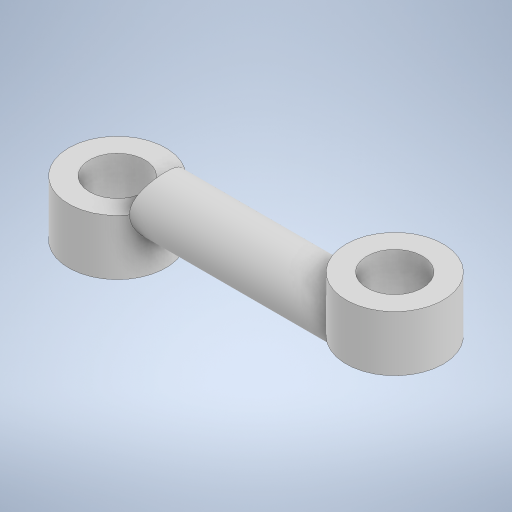
# Autodesk Inventor part: Part3
Saved by Autodesk Inventor 2024 (Build 280153000, 153)
## iProperties
Created: 2023-10-11
Part Number: Part3
Material: Generic
Document SubType Name: Modeling
Designer: owner
Density: 1 g/cm^3
Appearance: Default
Author: owner
Autodesk Inventor part; units mm, degrees
ref_plane "YZ Plane" through (0, 0, 0) normal (1, 0, 0) x (0, 1, 0)
ref_plane "XZ Plane" through (0, 0, 0) normal (0, 1, 0) x (-1, 0, 0)
ref_plane "XY Plane" through (0, 0, 0) normal (0, 0, 1) x (1, 0, 0)
sketch "Sketch1" plane through (0, 0, 0) normal (0, 0, 1) x (1, 0, 0)
  line L0 (-50, 0) -> (50, 0)
  line L1 (0, 0) -> (0, 34.9563) construction
  line L2 (-50, 0) -> (-50, 10)
  line L3 (-50, 10) -> (50, 10)
  line L4 (50, 10) -> (50, 0)
  dimension "d0" = 100
  dimension "d1" = 10
  constraints: 10 end point, 2 vertical, 1 horizontal, 1 midpoint, 1 parallel, 1 perpendicular
  measures "d0" distance of L0.start L0.end
  measures "d1" distance of L3.end L0.end
revolve "Revolution1" add sketch "Sketch1" angle 360 about axis through (-50, 0, 0) along (1, 0, 0)
sketch "Sketch2" plane through (0, 0, 0) normal (0, 1, 0) x (-1, 0, 0)
  line L0 (-50, 10) -> (-50, -10) projected
  circle A0 centre (-50, 0) radius 17.5
  circle A1 centre (-50, 0) radius 10
  point P0 (0, 0)
  dimension "d3" = 35
  dimension "d4" = 20
  constraints: 2 centre point, 1 coincident, 1 midpoint
  measures "d3" diameter of A0
  measures "d4" diameter of A1
extrude "Extrusion1" add sketch "Sketch2" along normal blind 20
extrude "Extrusion2" cut sketch "Sketch2" against normal blind 20 contours A1 L0 | A0 picked at (-47.9217, -2.6061)
extrude "Extrusion3" cut sketch "Sketch2" along normal blind 20 contours A1 L0 picked at (-47.9217, -2.6061)
sketch "Sketch4" plane through (0, 0, 0) normal (0, 1, 0) x (-1, 0, 0)
  line L0 (50, 10) -> (50, -10) projected
  circle A0 centre (50, 0) radius 17.5
  circle A1 centre (50, 0) radius 10
  point P0 (0, 0)
  dimension "d17" = 35
  dimension "d18" = 20
  constraints: 2 centre point, 1 coincident, 1 midpoint
  measures "d17" diameter of A0
  measures "d18" diameter of A1
extrude "Extrusion6" add sketch "Sketch4" against normal blind 20
extrude "Extrusion7" cut sketch "Sketch4" along normal blind 20 contours L0 A1 | A0 picked at (46.9919, -2.3982)
extrude "Extrusion8" cut sketch "Sketch4" against normal blind 20 contours L0 A1 picked at (46.9919, -2.3982)
body "Solid1"
